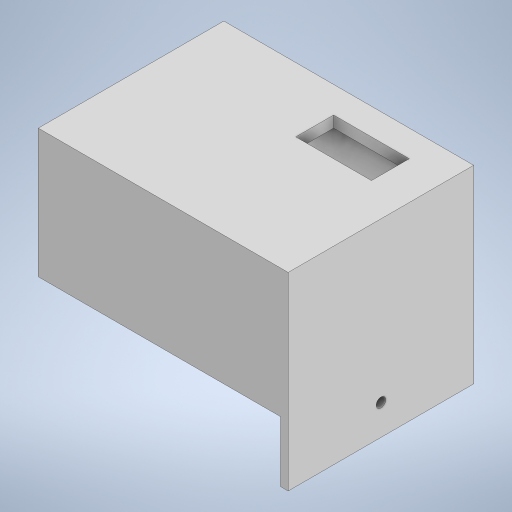
# Autodesk Inventor part: Back
Saved by Autodesk Inventor 2024 (Build 280153000, 153)
## iProperties
Created: 2023-12-18
Part Number: Back
Material: Generic
Document SubType Name: Modeling
Designer: Mechatronics Lab 1
Density: 1 g/cm^3
Appearance: Default
Author: Mechatronics Lab 1
Autodesk Inventor part; units mm, degrees
ref_plane "YZ Plane" through (0, 0, 0) normal (1, 0, 0) x (0, 1, 0)
ref_plane "XZ Plane" through (0, 0, 0) normal (0, 1, 0) x (-1, 0, 0)
ref_plane "XY Plane" through (0, 0, 0) normal (0, 0, 1) x (1, 0, 0)
sketch "Sketch94" plane through (0, 0, 0) normal (0, 1, 0) x (-1, 0, 0)
  line L0 (0, 0) -> (64, 0)
  line L1 (64, 0) -> (64, -49)
  line L2 (64, -49) -> (0, -49)
  line L3 (0, -49) -> (0, 0)
  dimension "d270" = 64
  dimension "d271" = 49
  constraints: 8 end point, 2 parallel, 1 horizontal, 1 perpendicular
  measures "d270" distance of L1.end L2.end
  measures "d271" distance of L0.end L1.end
extrude "Extrusion51" add sketch "Sketch94" along normal blind 3
sketch "Sketch96" plane through (0, 0, 0) normal (0, -1, 0) x (1, 0, 0)
  line L0 (-64, 0) -> (0, 0) projected
  line L1 (0, 0) -> (-64, 0)
  line L2 (-64, 0) -> (-64, -3)
  line L3 (-64, -49) -> (-64, 0) projected
  line L4 (-64, -3) -> (0, -3)
  line L5 (0, -3) -> (0, 0)
  dimension "d274" = 3
  constraints: 8 end point, 2 perpendicular, 1 collinear, 1 point on line
  measures "d274" distance of L0.start L2.end
extrude "Extrusion52" add sketch "Sketch96" along normal blind 31
sketch "Sketch97" plane through (0, 0, 0) normal (0, -1, 0) x (1, 0, 0)
  line L0 (0, -49) -> (-64, -49) projected
  line L1 (0, -49) -> (0, -46)
  line L2 (0, 0) -> (0, -49) projected
  line L3 (0, -46) -> (-64, -46)
  line L4 (-64, -49) -> (-64, 0) projected
  line L5 (-64, -49) -> (0, -49)
  dimension "d277" = 3
  constraints: 6 end point, 2 point on line, 1 parallel, 1 perpendicular
  measures "d277" distance of L0.start L1.end
extrude "Extrusion53" add sketch "Sketch97" along normal blind 31
sketch "Sketch98" plane through (0, 3, 0) normal (0, 1, 0) x (1, 0, 0)
  line L0 (-64, 49) -> (0, 49) projected
  line L1 (0, 49) -> (-8, 49)
  line L2 (-8, 49) -> (-8, 42)
  line L3 (-8, 42) -> (0, 42)
  line L4 (0, 42) -> (0, 49)
  line L5 (-8, 42) -> (-28, 42)
  line L6 (-28, 42) -> (-28, 32)
  line L7 (-28, 32) -> (-8, 32)
  line L8 (-8, 32) -> (-8, 42)
  point P0 (0, 0)
  dimension "d280" = 8
  dimension "d281" = 7
  dimension "d282" = 20
  dimension "d283" = 10
  constraints: 16 end point, 4 parallel, 2 horizontal, 2 perpendicular
  measures "d280" distance of L3.end L2.end
  measures "d281" distance of L2.end L1.end
  measures "d282" distance of L7.end L6.end
  measures "d283" distance of L6.end L5.end
extrude "Extrusion54" cut sketch "Sketch98" against normal blind 31 contours L8 L7 L6 L5
sketch "Sketch99" plane through (0, 3, 0) normal (0, 1, 0) x (1, 0, 0)
  line L0 (0, 0) -> (2, 0)
  line L1 (2, 0) -> (2, 49)
  line L2 (2, 49) -> (0, 49)
  line L3 (0, 49) -> (0, 0)
  dimension "d286" = 2
  dimension "d287" = 49
  constraints: 8 end point, 2 parallel, 1 horizontal, 1 perpendicular
  measures "d286" distance of L2.end L1.end
  measures "d287" distance of L1.end L0.end
extrude "Extrusion55" add sketch "Sketch99" against normal blind 50
sketch "Sketch100" plane through (0, 0, 0) normal (0, -1, 0) x (1, 0, 0)
  line L0 (-64, -46) -> (-64, -3) projected
  line L1 (-64, -3) -> (0, -3) projected
  line L2 (-64, -46) -> (-61, -46)
  line L3 (-61, -46) -> (-61, -3)
  line L4 (-61, -3) -> (-64, -3)
  line L5 (-64, -3) -> (-64, -46)
  point P0 (0, 0)
  dimension "d290" = 3
  constraints: 8 end point, 2 parallel, 1 horizontal, 1 perpendicular, 1 point on line
  measures "d290" distance of L4.end L3.end
extrude "Extrusion56" add sketch "Sketch100" along normal blind 13
sketch "Sketch101" plane through (2, 3, 0) normal (1, 0, 0) x (0, 0, -1)
  line L0 (0, -50) -> (49, -50) projected
  line L1 (0, -50) -> (24.5, -50)
  line L2 (24.5, -50) -> (24.5, -42)
  circle A0 centre (24.5, -42) radius 1.25
  point P0 (0, -3)
  dimension "d293" = 24.5
  dimension "d294" = 8
  dimension "d295" = 2.5
  constraints: 4 end point, 1 centre point, 1 coincident, 1 midpoint, 1 perpendicular
  measures "d293" distance of L0.start L1.end
  measures "d294" distance of L1.end L2.end
  measures "d295" diameter of A0
extrude "Extrusion57" cut sketch "Sketch101" against normal blind 13
body "Solid4"
